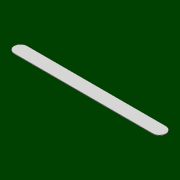
# Autodesk Inventor part: Part5
Saved by Autodesk Inventor 2018 (Build 220112000, 112)
## iProperties
Created: 2021-12-12
Part Number: Part5
Material: 一般
Document SubType Name: Modeling
Designer: gisen
Density: 1 g/cm^3
Appearance: 既定
Author: gisen
Autodesk Inventor part; units mm, degrees
ref_plane "YZ Plane" through (0, 0, 0) normal (1, 0, 0) x (0, 1, 0)
ref_plane "XZ Plane" through (0, 0, 0) normal (0, 1, 0) x (-1, 0, 0)
ref_plane "XY Plane" through (0, 0, 0) normal (0, 0, 1) x (1, 0, 0)
sketch "スケッチ1" plane through (0, 0, 0) normal (0, 0, 1) x (1, 0, 0)
  line L0 (0, 0) -> (274.4, 0) construction
  line L1 (0, -12.8) -> (274.4, -12.8)
  line L2 (274.4, 12.8) -> (0, 12.8)
  arc A0 (0, 12.8) -> (0, -12.8) centre (0, 0) ccw
  arc A1 (274.4, -12.8) -> (274.4, 12.8) centre (274.4, 0) ccw
  point P0 (137.2, 0)
  dimension "d0" = 274.4
  dimension "d2" = 25.6
  constraints: 8 end point, 4 point on circle, 4 tangent, 2 centre point, 1 horizontal, 1 midpoint, 1 parallel
  measures "d0" distance of L0.start L0.end
  measures "d2" distance between parallel lines of L1 L2
extrude "押し出し1" add sketch "スケッチ1" along normal blind 1
